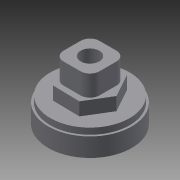
# Autodesk Inventor part: Top
Saved by Autodesk Inventor 2015 (Build 190159000, 159)
## iProperties
Created: 2015-02-14
Part Number: Top
Material: Generic
Document SubType Name: Modeling
Designer: chapale16
Density: 1 g/cm^3
Appearance: Default
Author: chapale16
Autodesk Inventor part; units mm, degrees
ref_plane "YZ Plane" through (0, 0, 0) normal (1, 0, 0) x (0, 1, 0)
ref_plane "XZ Plane" through (0, 0, 0) normal (0, 1, 0) x (-1, 0, 0)
ref_plane "XY Plane" through (0, 0, 0) normal (0, 0, 1) x (1, 0, 0)
sketch "Sketch1" plane through (0, 0, 0) normal (0, 1, 0) x (-1, 0, 0)
  circle A0 centre (0, 0) radius 28.3845
  circle A1 centre (0, 0) radius 6.35
  dimension "d0" = 56.769
  dimension "d1" = 12.7
  constraints: 2 centre point, 2 coincident
  measures "d0" diameter of A0
  measures "d1" diameter of A1
extrude "Extrusion1" add sketch "Sketch1" along normal blind 12.7
sketch "Sketch2" plane through (0, 12.7, 0) normal (0, 1, 0) x (1, 0, 0)
  circle A0 centre (0, 0) radius 26.9875
  circle A1 centre (0, 0) radius 6.35
  dimension "d4" = 53.975
  constraints: 2 centre point, 2 coincident
  measures "d4" diameter of A0
extrude "Extrusion2" add sketch "Sketch2" along normal blind 4.191
sketch "Sketch3" plane through (0, 16.891, 0) normal (0, 1, 0) x (1, 0, 0)
  line L0 (9.4957, 15.6943) -> (18.3395, -0.3764)
  line L1 (18.3395, -0.3764) -> (8.8438, -16.0707)
  line L2 (8.8438, -16.0707) -> (-9.4957, -15.6943)
  line L3 (-9.4957, -15.6943) -> (-18.3395, 0.3764)
  line L4 (-18.3395, 0.3764) -> (-8.8438, 16.0707)
  line L5 (-8.8438, 16.0707) -> (9.4957, 15.6943)
  circle A0 centre (0, 0) radius 6.35
  constraints: 12 end point, 2 coincident, 1 centre point, 13 other
extrude "Extrusion3" add sketch "Sketch3" along normal blind 8.89
sketch "Sketch4" plane through (0, 25.781, 0) normal (0, 1, 0) x (1, 0, 0)
  line L0 (-12.192, -12.192) -> (12.192, -12.192)
  line L1 (12.192, -12.192) -> (12.192, 12.192)
  line L2 (12.192, 12.192) -> (-12.192, 12.192)
  line L3 (-12.192, 12.192) -> (-12.192, -12.192)
  circle A0 centre (0, 0) radius 6.35
  dimension "d9" = 24.384
  dimension "d10" = 24.384
  constraints: 8 end point, 2 parallel, 1 centre point, 1 coincident, 1 horizontal, 1 perpendicular
  measures "d9" distance of L2.end L1.end
  measures "d10" distance of L1.end L0.end
extrude "Extrusion4" add sketch "Sketch4" along normal blind 14.224
fillet "Fillet1" radius 6.35 4 edges at (12.192, 32.893, 12.192) (12.192, 32.893, -12.192) (-12.192, 32.893, -12.192) (-12.192, 32.893, 12.192)
body "Solid1"
